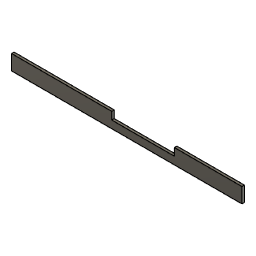
Bottom Rail v1 (Autodesk Fusion 360 design; units mm, degrees)
Autodesk Fusion 360 part; units mm, degrees
sketch "Sketch1" plane through (0, 0, 0) normal (0, 0, 1) x (1, 0, 0)
  line L0 (0, 19.05) -> (63.5, 19.05)
  line L1 (63.5, 19.05) -> (63.5, 9.525)
  line L2 (228.6, 0) -> (228.6, 19.05)
  line L3 (142.875, 19.05) -> (142.875, 9.525)
  line L4 (0, 0) -> (228.6, 0)
  line L5 (63.5, 9.525) -> (142.875, 9.525)
  line L6 (228.6, 19.05) -> (142.875, 19.05)
  line L7 (0, 19.05) -> (-63.5, 19.05)
  line L8 (-63.5, 19.05) -> (-63.5, 0)
  line L9 (-63.5, 0) -> (0, 0)
  dimension "d7" = 228.6
  dimension "d8" = 19.05
  dimension "d9" = 19.05
  dimension "d10" = 63.5
  dimension "d16" = 9.525
  dimension "d17" = 9.525
  dimension "d13" = 63.5
  constraint coincident L4.start L9.end
  constraint horizontal L4
  constraint perpendicular L2 L4
  constraint perpendicular L2 L6
  constraint perpendicular L0 L1
  constraint perpendicular L3 L6
  constraint parallel L0 L7
  constraint perpendicular L7 L8
  constraint perpendicular L8 L9
  measures "d7" distance of L2.start L4.start
  measures "d8" distance of L4.start L0.start
  measures "d9" distance of L2.start L2.end
  measures "d10" distance of L0.end L0.start
  measures "d16" distance of L1.end L0.end
  measures "d17" distance of L3.end L3.start
  measures "d13" distance of L0.start L7.end
extrude "Extrude1" add sketch "Sketch1" along normal blind 3.175
equation "d7 = 9\""
equation "d8 = ( 3 / 4 ) * 1 in"
equation "d9 = ( 3 / 4 ) * 1 in"
equation "d16 = ( 3 / 8 ) * 1 in"
